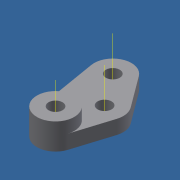
# Autodesk Inventor part: 3_hebenMount_2_dual
Saved by Autodesk Inventor 2016 (Build 200138000, 138)
## iProperties
Created: 2014-12-28
Part Number: 3_hebenMount_2_dual
Material: Generisch
Document SubType Name: Modeling
Designer: 4ndreas
Density: 1 g/cm^3
Appearance: Vorgabe
Mass: 0.666131 g
Surface Area: 7.15227 cm^2
Volume: 0.666131 cm^3
Author: 4ndreas
Autodesk Inventor part; units mm, degrees
ref_plane "YZ Plane" through (0, 0, 0) normal (1, 0, 0) x (0, 1, 0)
ref_plane "XZ Plane" through (0, 0, 0) normal (0, 1, 0) x (-1, 0, 0)
ref_plane "XY Plane" through (0, 0, 0) normal (0, 0, 1) x (1, 0, 0)
sketch "Skizze1" plane through (0, 0, 0) normal (0, 0, 1) x (1, 0, 0)
  circle A0 centre (0, 0) radius 4
  circle A1 centre (-2.5, 14.7902) radius 1.5
  circle A2 centre (2.5, 8.029) radius 1.5
  line L0 (-4, 0) -> (-4, 14.7902)
  line L1 (-1.294, 15.6821) -> (3.706, 8.9208)
  line L2 (4, 8.029) -> (4, 0)
  line L3 (0, 0) -> (-2.5, 14.7902) construction
  line L4 (2.5, 8.029) -> (-1.25, 7.3951) construction
  dimension "d0" = 8
  dimension "d1" = 3
  dimension "d3" = 15
  constraints: 10 end point, 6 point on circle, 6 tangent, 3 centre point, 2 coincident, 1 equal radius, 1 midpoint, 1 parallel, 1 perpendicular, 1 vertical
  measures "d0" diameter of A0
  measures "d1" diameter of A1
  measures "d3" distance of L3.end point (0, 0)
extrude "Extrusion1" add sketch "Skizze1" along normal blind 3
sketch "Skizze2" plane through (0, 0, 3) normal (0, 0, 1) x (1, 0, 0)
  arc A0 (4, 8.029) -> (3.706, 8.9208) centre (2.5, 8.029) ccw projected
  arc A1 (-1.294, 15.6821) -> (-4, 14.7902) centre (-2.5, 14.7902) ccw projected
  arc A2 (-4, 0) -> (4, 0) centre (0, 0) ccw projected
hole "Bohrung1" at (2.5, 8.029, 3) at (-2.5, 14.7902, 3) at (0, 0, 3) direction (0, 0, -1) diameter 3 end through all
sketch "Skizze3" plane through (0, 0, 3) normal (0, 0, 1) x (1, 0, 0)
  circle A0 centre (-2.5, 14.7902) radius 1.5 projected
  circle A1 centre (2.5, 8.029) radius 1.5 projected
  arc A2 (4, 8.029) -> (3.706, 8.9208) centre (2.5, 8.029) ccw projected
  line L0 (3.706, 8.9208) -> (-1.294, 15.6821) projected
  arc A3 (-1.294, 15.6821) -> (-4, 14.7902) centre (-2.5, 14.7902) ccw projected
  line L1 (-4, 14.7902) -> (-4, 0) projected
  arc A4 (-4, 0) -> (4, 0) centre (0, 0) ccw projected
  line L2 (4, 0) -> (4, 8.029) projected
  arc A5 (0.7161, 17.1686) -> (-6.4441, 14.1235) centre (-2.5, 14.7902) ccw
  arc A6 (6.3191, 6.8398) -> (5.7161, 10.4073) centre (2.5, 8.029) ccw
  arc A7 (-3.9441, -0.6667) -> (3.8191, -1.1892) centre (0, 0) ccw
  line L3 (3.8191, -1.1892) -> (6.3191, 6.8398)
  line L4 (-3.9441, -0.6667) -> (-6.4441, 14.1235)
  line L5 (0.7161, 17.1686) -> (5.7161, 10.4073)
  circle A8 centre (0, 0) radius 1.5 projected
  dimension "d13" = 2.5
  dimension "d14" = 2.5
  dimension "d24" = 2.5
  constraints: 7 tangent, 6 end point, 6 point on circle, 3 centre point, 3 coincident
  measures "d13" radial gap between concentric circles of A5 A0
  measures "d14" radial gap between concentric circles of A6 A1
  measures "d24" radial gap between concentric circles of A4 A8
extrude "Extrusion2" add sketch "Skizze3" against normal up to surface (3 mm away) contours A0 L1 A4 L4 A5 L5 A6 L3 L2 A1 L0
sketch "Skizze4" plane through (0, 0, 3) normal (0, 0, 1) x (1, 0, 0)
  arc A0 (6.3191, 6.8398) -> (5.7161, 10.4073) centre (2.5, 8.029) ccw projected
  arc A1 (0.7161, 17.1686) -> (-6.4441, 14.1235) centre (-2.5, 14.7902) ccw projected
  arc A2 (0.2281, 11.8649) -> (-0.5021, 11.3249) centre (2.5, 8.029) ccw
  arc A3 (0.2281, 11.8649) -> (0.7161, 17.1686) centre (-2.5, 14.7902) ccw
  arc A4 (-6.4441, 14.1235) -> (-0.5021, 11.3249) centre (-2.5, 14.7902) ccw
  circle A5 centre (2.5, 8.029) radius 1.5 projected
  arc A6 (-3.9441, -0.6667) -> (3.8191, -1.1892) centre (0, 0) ccw projected
  arc A7 (0.2261, 3.9936) -> (2.081, 3.416) centre (0, 0) ccw
  arc A8 (0.2261, 3.9936) -> (2.081, 3.416) centre (2.5, 8.029) ccw
  circle A9 centre (0, 0) radius 1.5 projected
  constraints: 10 point on circle, 5 centre point, 5 coincident, 1 concentric
extrude "Extrusion3" add sketch "Skizze4" along normal blind 2.6 contours A7 A8 A6
equation "\"d0\" = 2 * bearingWall"
equation "\"d1\" = bearingHole"
equation "\"d3\" = Hebel_basis_2"
equation "\"d4\" = Join_width"
equation "\"d6\" = bearingHole"
equation "\"d13\" = d24"
equation "\"d14\" = d13"
equation "\"FingerLaenge_B\" = 25"
equation "\"Hebel_B\" = 25"
equation "\"Finger_width\" = 22"
equation "\"Finger_diameter\" = 8"
equation "\"FingerWall\" = 3"
equation "\"Hebel_basis_2\" = 15"
equation "\"Join_width\" = 3"
equation "\"bearingHole\" = 3"
equation "\"bearingWall\" = 4"
equation "\"support_D\" = 0.25"
